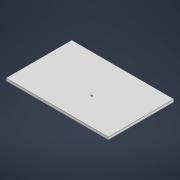
# Autodesk Inventor part: holder3_l1
Saved by Autodesk Inventor 2021 (Build 250183000, 183)
## iProperties
Created: 2021-06-13
Part Number: holder3_l1
Material: Generic
Document SubType Name: Modeling
Designer: Watchdog
Density: 1 g/cm^3
Appearance: Default
Author: Watchdog
Autodesk Inventor part; units mm, degrees
ref_plane "YZ Plane" through (0, 0, 0) normal (1, 0, 0) x (0, 1, 0)
ref_plane "XZ Plane" through (0, 0, 0) normal (0, 1, 0) x (-1, 0, 0)
ref_plane "XY Plane" through (0, 0, 0) normal (0, 0, 1) x (1, 0, 0)
sketch "Sketch1" plane through (0, 0, 0) normal (0, 1, 0) x (-1, 0, 0)
  line L0 (215.3593, -148.8302) -> (-182.955, -148.8302)
  line L1 (-182.955, -148.8302) -> (-182.955, 106.9627)
  line L2 (-182.955, 106.9627) -> (215.3593, 106.9627)
  line L3 (215.3593, 106.9627) -> (215.3593, -148.8302)
  point P0 (0, 0)
  constraints: 8 end point, 2 parallel, 1 horizontal, 1 perpendicular
extrude "Extrusion1" add sketch "Sketch1" along normal blind 10
sketch "Sketch2" plane through (0, 10, 0) normal (0, 1, 0) x (1, 0, 0)
  point P0 (0, 0)
  point P1 (12.113, 0)
  dimension "d2" = 12.113
  measures "d2" distance of point (0, 0) point (12.113, 0)
hole "Hole1" at (12.113, 10, 0) direction (0, -1, 0) diameter 6 end through all
body "Solid1"
